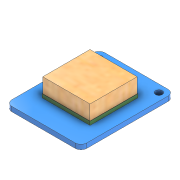
# Autodesk Inventor part: GPS
Saved by Autodesk Inventor 2022.3 (Build 263350000, 350)
## iProperties
Created: 2023-07-31
Part Number: GPS
Material: Genérico
Document SubType Name: Modeling
Designer: Usuario
Density: 1 g/cm^3
Appearance: Valor por defecto
Author: Usuario
Autodesk Inventor part; units mm, degrees
ref_plane "YZ Plane" through (0, 0, 0) normal (1, 0, 0) x (0, 1, 0)
ref_plane "XZ Plane" through (0, 0, 0) normal (0, 1, 0) x (-1, 0, 0)
ref_plane "XY Plane" through (0, 0, 0) normal (0, 0, 1) x (1, 0, 0)
sketch "Boceto1" plane through (0, 0, 0) normal (0, 1, 0) x (-1, 0, 0)
  line L0 (-10.7, 15.75) -> (10.7, 15.75)
  line L1 (12.7, 13.75) -> (12.7, -13.75)
  line L2 (10.7, -15.75) -> (-10.7, -15.75)
  line L3 (-12.7, -13.75) -> (-12.7, 13.75)
  line L4 (-12.7, 15.75) -> (12.7, -15.75) construction
  line L5 (12.7, 15.75) -> (-12.7, -15.75) construction
  arc A0 (10.7, -15.75) -> (12.7, -13.75) centre (10.7, -13.75) ccw
  arc A1 (12.7, 13.75) -> (10.7, 15.75) centre (10.7, 13.75) ccw
  arc A2 (-10.7, 15.75) -> (-12.7, 13.75) centre (-10.7, 13.75) ccw
  arc A3 (-12.7, -13.75) -> (-10.7, -15.75) centre (-10.7, -13.75) ccw
  line L6 (0, -15.75) -> (0, -13.21)
  line L7 (0, -13.21) -> (10.16, -13.21)
  line L8 (0, -13.21) -> (-10.16, -13.21)
  circle A4 centre (10.16, -13.21) radius 1.15
  circle A5 centre (-10.16, -13.21) radius 1.15
  point P0 (0, 0)
  dimension "d0" = 25.4
  dimension "d1" = 31.5
  dimension "d2" = 2
  dimension "d3" = 2.54
  dimension "d4" = 10.16
  dimension "d5" = 10.16
  dimension "d6" = 2.3
  dimension "d7" = 2.3
  constraints: 18 end point, 8 point on circle, 8 point on line, 8 tangent, 6 centre point, 3 equal radius, 3 horizontal, 3 midpoint, 2 coincident, 2 parallel, 1 perpendicular, 1 vertical
  measures "d0" distance of L4.end L5.end
  measures "d1" distance of L5.start L4.end
  measures "d2" radius of A0
  measures "d3" distance of L6.start L6.end
  measures "d4" distance of L6.end L7.end
  measures "d5" distance of L6.end L8.end
  measures "d6" diameter of A4
  measures "d7" diameter of A5
extrude "Extrusión1" add sketch "Boceto1" along normal blind 1.6
sketch "Boceto2" plane through (0, 1.6, 0) normal (0, 1, 0) x (1, 0, 0)
  line L0 (-8, -8) -> (8, -8)
  line L1 (8, -8) -> (8, 8)
  line L2 (8, 8) -> (-8, 8)
  line L3 (-8, 8) -> (-8, -8)
  line L4 (-8, -8) -> (8, 8) construction
  line L5 (8, -8) -> (-8, 8) construction
  point P0 (0, 0)
  dimension "d10" = 16
  dimension "d11" = 16
  constraints: 12 end point, 2 midpoint, 2 parallel, 1 horizontal, 1 perpendicular
  measures "d10" distance of L2.end L1.end
  measures "d11" distance of L1.end L0.end
extrude "Extrusión2" add sketch "Boceto2" along normal blind 6.2
sketch "Boceto3" plane through (0, 1.6, 0) normal (0, 1, 0) x (1, 0, 0)
  line L0 (8.1, -8.1) -> (-8.1, -8.1)
  line L1 (-8.1, -8.1) -> (-8.1, 8.1)
  line L2 (-8.1, 8.1) -> (8.1, 8.1)
  line L3 (8.1, 8.1) -> (8.1, -8.1)
  line L4 (8.1, -8.1) -> (-8.1, 8.1) construction
  line L5 (-8.1, -8.1) -> (8.1, 8.1) construction
  point P0 (0, 0)
  dimension "d14" = 16.2
  dimension "d15" = 16.2
  constraints: 12 end point, 2 midpoint, 2 parallel, 1 horizontal, 1 perpendicular
  measures "d14" distance of L1.end L2.end
  measures "d15" distance of L0.end L1.end
extrude "Extrusión3" add sketch "Boceto3" along normal blind 1.2
